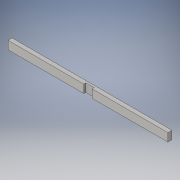
# Autodesk Inventor part: Cabinet Support Frame Horizontal Bar Low
Saved by Autodesk Inventor 2016 (Build 200138000, 138)
## iProperties
Created: 2018-01-15
Part Number: Cabinet Support Frame Horizontal Bar Low
Material: Generic
Document SubType Name: Modeling
Designer: dash
Density: 1 g/cm^3
Appearance: Default
Author: dash
Autodesk Inventor part; units mm, degrees
ref_plane "YZ Plane" through (0, 0, 0) normal (1, 0, 0) x (0, 1, 0)
ref_plane "XZ Plane" through (0, 0, 0) normal (0, 1, 0) x (-1, 0, 0)
ref_plane "XY Plane" through (0, 0, 0) normal (0, 0, 1) x (1, 0, 0)
sketch "Sketch1" plane through (0, 0, 0) normal (0, 0, 1) x (1, 0, 0)
  line L0 (0, 0) -> (742.95, 0)
  line L1 (742.95, 0) -> (742.95, 38.1)
  line L2 (742.95, 38.1) -> (0, 38.1)
  line L3 (0, 38.1) -> (0, 0)
  dimension "d0" = 742.95
  dimension "d1" = 38.1
  constraints: 8 end point, 2 parallel, 1 horizontal, 1 perpendicular
  measures "d0" distance of L2.end L1.end
  measures "d1" distance of L1.end L0.end
extrude "Board" add sketch "Sketch1" along normal blind 19.05
sketch "Sketch2" plane through (0, 0, 19.05) normal (0, 0, 1) x (1, 0, 0)
  line L0 (742.95, 38.1) -> (0, 38.1) projected
  line L1 (0, 0) -> (742.95, 0) projected
  line L2 (352.425, 38.1) -> (390.525, 38.1)
  line L3 (390.525, 38.1) -> (390.525, 0)
  line L4 (390.525, 0) -> (352.425, 0)
  line L5 (352.425, 0) -> (352.425, 38.1)
  line L6 (0, 38.1) -> (0, 0) projected
  dimension "d4" = 38.1
  dimension "d5" = 352.425
  constraints: 8 end point, 2 parallel, 2 point on line, 1 horizontal, 1 perpendicular
  measures "d4" distance of L3.end L4.end
  measures "d5" distance between parallel lines of L6 L5
extrude "Extrusion2" cut sketch "Sketch2" against normal blind 9.525 contours L3 L1 L5 L0
equation "\"d5\" = -0.5 * d4 + 0.5 * d0"
body "Solid1"
